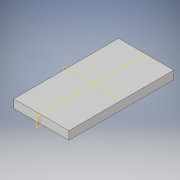
# Autodesk Inventor part: rev1 top
Saved by Autodesk Inventor 2017 (Build 210142000, 142)
## iProperties
Created: 2019-05-04
Part Number: rev1 top
Material: Generic
Document SubType Name: Modeling
Designer: Roman
Density: 1 g/cm^3
Appearance: Default
Author: Roman
Autodesk Inventor part; units mm, degrees
ref_plane "YZ Plane" through (0, 0, 0) normal (1, 0, 0) x (0, 1, 0)
ref_plane "XZ Plane" through (0, 0, 0) normal (0, 1, 0) x (-1, 0, 0)
ref_plane "XY Plane" through (0, 0, 0) normal (0, 0, 1) x (1, 0, 0)
sketch "Sketch1" plane through (0, 0, 0) normal (0, 1, 0) x (-1, 0, 0)
  line L0 (0, 0) -> (-1016, 0)
  line L1 (-1016, 0) -> (-1016, -1930.4)
  line L2 (-1016, -1930.4) -> (0, -1930.4)
  line L3 (0, -1930.4) -> (0, 0)
  dimension "d0" = 1016
  dimension "d1" = 1930.4
  constraints: 8 end point, 2 parallel, 1 horizontal, 1 perpendicular
  measures "d0" distance of L2.end L1.end
  measures "d1" distance of L1.end L0.end
extrude "Extrusion1" add sketch "Sketch1" against normal blind 152.4
sketch "Sketch2" plane through (0, -152.4, 0) normal (0, -1, 0) x (1, 0, 0)
  line L0 (25.4, -25.4) -> (990.6, -25.4)
  line L1 (990.6, -25.4) -> (990.6, -1905)
  line L2 (990.6, -1905) -> (25.4, -1905)
  line L3 (25.4, -1905) -> (25.4, -25.4)
  line L4 (25.4, -965.2) -> (0, -965.2)
  line L5 (0, 0) -> (0, -1930.4) projected
  line L6 (508, -1905) -> (508, -1930.4)
  line L7 (0, -1930.4) -> (1016, -1930.4) projected
  line L8 (990.6, -965.2) -> (1016, -965.2)
  line L9 (1016, -1930.4) -> (1016, 0) projected
  line L10 (508, -25.4) -> (508, 0)
  line L11 (1016, 0) -> (0, 0) projected
  dimension "d4" = 25.4
  dimension "d5" = 25.4
  constraints: 16 end point, 8 midpoint, 2 collinear, 2 parallel, 1 horizontal, 1 perpendicular
  measures "d4" distance of L4.start L4.end
  measures "d5" distance of L10.start L10.end
extrude "Extrusion2" cut sketch "Sketch2" against normal blind 50.8 contours L0 L1 L2 L3
sketch "Sketch3" plane through (0, -101.6, 0) normal (0, -1, 0) x (1, 0, 0)
  line L0 (990.6, -25.4) -> (990.6, -1905) projected
  line L1 (990.6, -279.4) -> (965.2, -279.4)
  line L2 (965.2, -279.4) -> (965.2, -736.6)
  line L3 (965.2, -736.6) -> (990.6, -736.6)
  line L4 (990.6, -736.6) -> (990.6, -279.4)
  line L5 (25.4, -1905) -> (25.4, -25.4) projected
  line L6 (990.6, -1905) -> (25.4, -1905) projected
  line L7 (990.6, -25.4) -> (990.6, -1905) projected
  line L8 (25.4, -25.4) -> (990.6, -25.4) projected
  line L9 (990.6, -1651) -> (965.2, -1651)
  line L10 (965.2, -1651) -> (965.2, -1193.8)
  line L11 (965.2, -1193.8) -> (990.6, -1193.8)
  line L12 (990.6, -1193.8) -> (990.6, -1651)
  point P0 (0, 0)
  dimension "d8" = 25.4
  dimension "d9" = 457.2
  dimension "d10" = 254
  dimension "d11" = 25.4
  dimension "d12" = 457.2
  dimension "d13" = 254
  constraints: 16 end point, 4 parallel, 2 horizontal, 2 perpendicular, 2 point on line
  measures "d8" distance of L3.end L2.end
  measures "d9" distance of L2.end L1.end
  measures "d10" distance between parallel lines of L8 L1
  measures "d11" distance of L10.end L11.end
  measures "d12" distance of L9.end L10.end
  measures "d13" distance between parallel lines of L6 L9
extrude "Extrusion3" cut sketch "Sketch3" against normal blind 50.8 contours L0 L3 L2 L1 | L0 L9 L10 L11
ref_plane "Work Plane1" through (508, 0, 0) normal (1, 0, 0) x (0, 0, -1)
mirror "Mirror1" about plane through (508, 0, 0) normal (1, 0, 0) of "Extrusion3"
sketch "Sketch4" plane through (0, -101.6, 0) normal (0, -1, 0) x (1, 0, 0)
  line L0 (25.4, -25.4) -> (990.6, -25.4) projected
  line L1 (812.8, -25.4) -> (660.4, -25.4)
  line L2 (660.4, -25.4) -> (660.4, -50.8)
  line L3 (660.4, -50.8) -> (812.8, -50.8)
  line L4 (812.8, -50.8) -> (812.8, -25.4)
  line L5 (355.6, -25.4) -> (203.2, -25.4)
  line L6 (203.2, -25.4) -> (203.2, -50.8)
  line L7 (203.2, -50.8) -> (355.6, -50.8)
  line L8 (355.6, -50.8) -> (355.6, -25.4)
  line L9 (990.6, -25.4) -> (990.6, -1905) projected
  line L10 (25.4, -1905) -> (25.4, -25.4) projected
  point P0 (0, 0)
  dimension "d16" = 152.4
  dimension "d17" = 25.4
  dimension "d18" = 152.4
  dimension "d19" = 25.4
  dimension "d20" = 177.8
  dimension "d21" = 177.8
  constraints: 16 end point, 4 parallel, 2 horizontal, 2 perpendicular, 2 point on line
  measures "d16" distance of L3.end L2.end
  measures "d17" distance of L2.end L1.end
  measures "d18" distance of L7.end L6.end
  measures "d19" distance of L6.end L5.end
  measures "d20" distance between parallel lines of L9 L4
  measures "d21" distance between parallel lines of L10 L6
extrude "Extrusion4" cut sketch "Sketch4" against normal blind 50.8
ref_plane "Work Plane2" through (0, 0, -965.2) normal (0, 0, 1) x (1, 0, 0)
mirror "Mirror2" about plane through (0, 0, -965.2) normal (0, 0, 1) of "Extrusion4"
body "Solid1"
